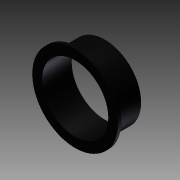
# Autodesk Inventor part: 80F-5020
Saved by Autodesk Inventor 2011 SP1 (Build 150282100, 282)
## iProperties
Created: 2011-08-31
Part Number: 80F-5020
Document SubType Name: Modeling
Designer: arihon
Density: 1 g/cm^3
Author: arihon
Autodesk Inventor part; units mm, degrees
ref_plane "YZ Plane" through (0, 0, 0) normal (1, 0, 0) x (0, 1, 0)
ref_plane "XZ Plane" through (0, 0, 0) normal (0, 1, 0) x (-1, 0, 0)
ref_plane "XY Plane" through (0, 0, 0) normal (0, 0, 1) x (1, 0, 0)
sketch "スケッチ1" plane through (0, 0, 0) normal (0, 0, 1) x (1, 0, 0)
  line L0 (0, 0) -> (0, 21.2524)
  line L1 (-27.5, 20) -> (-25.1, 20)
  line L2 (-25.1, 20) -> (-25.1, 0)
  line L3 (-25.1, 0) -> (-27.5, 0)
  line L4 (-27.5, 0) -> (-27.5, 20)
  line L5 (-25.1, 0) -> (-32.5, 0)
  line L6 (-32.5, 0) -> (-32.5, -2.5)
  line L7 (-32.5, -2.5) -> (-25.1, -2.5)
  line L8 (-25.1, -2.5) -> (-25.1, 0)
  dimension "d0" = 55
  dimension "d1" = 50.2
  dimension "d2" = 20
  dimension "d3" = 2.5
  dimension "d4" = 65
  constraints: 18 end point, 4 parallel, 2 horizontal, 2 perpendicular, 1 vertical
  measures "d0" diameter of L4 L0
  measures "d1" diameter of L2 L0
  measures "d2" distance of L3.end L1.start
  measures "d3" distance of L5.end L6.end
  measures "d4" diameter of L6 L0
revolve "回転1" add sketch "スケッチ1" angle 360 about axis through (0, 0, 0) along (0, 1, 0)
